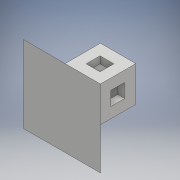
# Autodesk Inventor part: frame_nexus_2_base
Saved by Autodesk Inventor 2017 (Build 210142000, 142)
## iProperties
Created: 2017-01-29
Part Number: frame_nexus_2_base
Material: Generic
Document SubType Name: Modeling
Designer: Gabe Madonna
Density: 1 g/cm^3
Appearance: Default
Author: Gabe Madonna
Autodesk Inventor part; units mm, degrees
ref_plane "YZ Plane" through (0, 0, 0) normal (1, 0, 0) x (0, 1, 0)
ref_plane "XZ Plane" through (0, 0, 0) normal (0, 1, 0) x (-1, 0, 0)
ref_plane "XY Plane" through (0, 0, 0) normal (0, 0, 1) x (1, 0, 0)
sketch "Sketch1" plane through (0, 0, 0) normal (0, 1, 0) x (-1, 0, 0)
  line L0 (-12.7, -12.7) -> (-12.7, 12.7)
  line L1 (-12.7, 12.7) -> (12.7, 12.7)
  line L2 (12.7, 12.7) -> (12.7, -12.7)
  line L3 (12.7, -12.7) -> (-12.7, -12.7)
  point P0 (0, 0)
  point P1 (0, 0)
  dimension "d0" = 25.4
  constraints: 8 end point, 1 coincident, 9 other
  measures "d0" distance of L1.end L2.end
extrude "Extrusion1" add sketch "Sketch1" along normal blind 25.4
sketch "Sketch2" plane through (0, 25.4, 0) normal (0, 1, 0) x (1, 0, 0)
  line L0 (9.525, 9.525) -> (9.525, -9.525)
  line L1 (9.525, -9.525) -> (-9.525, -9.525)
  line L2 (-9.525, -9.525) -> (-9.525, 9.525)
  line L3 (-9.525, 9.525) -> (9.525, 9.525)
  point P0 (0, 0)
  point P1 (0, 0)
  dimension "d3" = 19.05
  constraints: 8 end point, 1 coincident, 9 other
  measures "d3" distance of L1.end L2.end
extrude "Extrusion2" cut sketch "Sketch2" against normal blind 5
sketch "Sketch3" plane through (12.7, 0, 12.7) normal (1, 0, 0) x (0, 0, -1)
  line L0 (22.225, 20.4) -> (3.175, 20.4) projected
  line L1 (17.7, 7.4) -> (7.7, 7.4)
  line L2 (7.7, 7.4) -> (7.7, 17.4)
  line L3 (7.7, 17.4) -> (17.7, 17.4)
  line L4 (17.7, 17.4) -> (17.7, 7.4)
  point P0 (12.7, 0)
  point P1 (12.7, 12.4)
  dimension "d6" = 10
  constraints: 8 end point, 9 other
  measures "d6" distance of L1.start L1.end
extrude "Extrusion3" cut sketch "Sketch3" against normal blind 5
pattern_circular "Circular Pattern1" count 4 over 360 about axis through (0, -10, 0) along (0, 1, 0) of "Extrusion3"
sketch "Sketch4" plane through (0, 0, 0) normal (0, -1, 0) x (1, 0, 0)
  line L0 (12.7, -12.7) -> (12.7, 12.7) projected
  line L1 (12.7, 12.7) -> (-12.7, 12.7) projected
  line L2 (-12.7, 12.7) -> (-12.7, -12.7) projected
  line L3 (-12.7, -12.7) -> (12.7, -12.7) projected
  point P0 (0, 0)
extrude "Extrusion4" add sketch "Sketch4" along normal blind 15 draft 45
body "Solid1"
